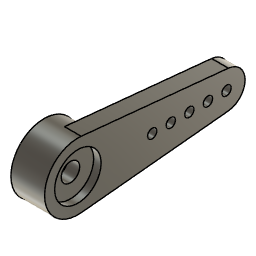
Servo half arm v1 (Autodesk Fusion 360 design; units mm, degrees)
Autodesk Fusion 360 part; units mm, degrees
note: some values were not read from the file. Set by a fixed rule: which sketch regions a step uses.
sketch "Sketch1" plane through (0, 0, 0) normal (1, 0, 0) x (0, 1, 0)
  circle A0 centre (0, 0) radius 3.58
  circle A1 centre (16, 0) radius 2
  line L0 (0.3535, 3.5625) -> (16.1975, 1.9902)
  line L1 (0.3535, -3.5625) -> (16.1975, -1.9902)
  circle A2 centre (16, 0) radius 0.5
  circle A3 centre (14, 0) radius 0.5
  circle A4 centre (12, 0) radius 0.5
  circle A5 centre (10, 0) radius 0.5
  circle A6 centre (8, 0) radius 0.5
  line L2 (0, 7) -> (0, -7.5)
  circle A7 centre (-8, 0) radius 0.5
  circle A8 centre (-10, 0) radius 0.5
  line L3 (-0.3535, 3.5625) -> (-16.1975, 1.9902)
  circle A9 centre (-12, 0) radius 0.5
  circle A10 centre (-14, 0) radius 0.5
  circle A11 centre (-16, 0) radius 2
  circle A12 centre (-16, 0) radius 0.5
  line L4 (-0.3535, -3.5625) -> (-16.1975, -1.9902)
  dimension "d4" = 7.16
  dimension "d5" = 4
  dimension "d6" = 16
  dimension "d7" = 1
  dimension "d10" = -8
  dimension "d11" = 0
  constraint coincident A0.centre origin
  constraint coincident A0 L0.start
  constraint coincident A1 L0.end
  constraint coincident A0 L1.start
  constraint coincident A1 L1.end
  constraint tangent A0 L0
  constraint tangent A1 L0
  constraint tangent A1 L1
  constraint tangent A0 L1
  constraint concentric A1 A2
  constraint vertical L2
  constraint coincident A0.centre L2
  constraint symmetric A1 L2 A11
  constraint symmetric L0.start L2 L3.start
  constraint symmetric L0.end L2 L3.end
  constraint symmetric L1.start L2 L4.start
  constraint symmetric L1.end L2 L4.end
  constraint symmetric A2 L2 A12
  constraint symmetric A3 L2 A10
  constraint symmetric A4 L2 A9
  constraint symmetric A5 L2 A8
  constraint symmetric A6 L2 A7
  measures "d4" diameter of A0
  measures "d5" diameter of A1
  measures "d6" distance of A0.centre A1.centre
  measures "d7" diameter of A2
extrude "Extrude1" add sketch "Sketch1" along normal blind 1.8 contours A0 L2 | A0 A1 L0 L1 A3 | A0 L2 | A1 A3 | A0 L3 A10 A11 L4 | A10 A11 picked at (14.8153, -0.6023) picked at (-14.8153, -0.6023) makes body 1
extrude "Extrude2" add sketch "Sketch1" along normal blind 1.8 separate body contours A0 L2 | A0 A1 L0 L1 A3 | A0 L2 | A1 A3 picked at (14.8153, -0.6023) makes body 2
sketch "Sketch2" plane through (0, 0, 0) normal (1, 0, 0) x (0, 1, 0)
extrude "Extrude3" add sketch "Sketch1" against normal blind 1.83 contours A0 L2 | A0 L2 bodies 1
sketch "Sketch3" plane through (1.8, 0, 0) normal (1, 0, 0) x (0, 1, 0)
  circle A0 centre (-10, 0) radius 0.5
  circle A1 centre (10, 0) radius 0.5
  circle A2 centre (-12, 0) radius 0.5
  circle A3 centre (12, 0) radius 0.5
  circle A4 centre (-8, 0) radius 0.5
  circle A5 centre (16, 0) radius 0.5
  circle A6 centre (-16, 0) radius 0.5
  circle A7 centre (14, 0) radius 0.5
  circle A8 centre (8, 0) radius 0.5
  circle A9 centre (-14, 0) radius 0.5
  line L0 (0.3535, -3.5625) -> (16.1975, -1.9902)
  arc A10 (16.1975, -1.9902) -> (16.1975, 1.9902) centre (16, 0) ccw
  line L1 (16.1975, 1.9902) -> (0.3535, 3.5625)
  arc A11 (0.3535, 3.5625) -> (-0.3535, 3.5625) centre (0, 0) ccw
  line L2 (-0.3535, 3.5625) -> (-16.1975, 1.9902)
  arc A12 (-16.1975, 1.9902) -> (-16.1975, -1.9902) centre (-16, 0) ccw
  line L3 (-16.1975, -1.9902) -> (-0.3535, -3.5625)
  arc A13 (-0.3535, -3.5625) -> (0.3535, -3.5625) centre (0, 0) ccw
  circle A14 centre (0, 0) radius 2.5
  circle A15 centre (0, 0) radius 3.58
  dimension "d18" = 5
  constraint concentric A14 A15
  measures "d18" diameter of A14
extrude "Extrude4" cut sketch "Sketch3" against normal blind 0.8 contours A14 bodies 1
sketch "Sketch4" plane through (1, 0, 0) normal (1, 0, 0) x (0, 1, 0)
  circle A0 centre (0, 0) radius 2.5
  circle A1 centre (0, 0) radius 2.5
  circle A2 centre (0, 0) radius 1
  dimension "d21" = 2
  constraint concentric A0 A1
  constraint concentric A1 A2
  measures "d21" diameter of A2
extrude "Extrude5" cut sketch "Sketch4" against normal blind 13.5 contours A2 bodies 1
sketch "Sketch5" plane through (-1.83, 0, 0) normal (-1, 0, 0) x (0, -1, 0)
  circle A0 centre (0, 0) radius 1
  circle A1 centre (0, 0) radius 3.58
  circle A2 centre (0, 0) radius 2.3
  dimension "d24" = 4.6
  constraint concentric A0 A2
  measures "d24" diameter of A2
extrude "Extrude6" cut sketch "Sketch5" against normal blind 1.5 contours A2 bodies 1
extrude "Extrude7" add sketch "Sketch1" against normal blind 1.83 contours A0 L2 | A0 L2 bodies 2
extrude "Extrude8" cut sketch "Sketch3" against normal blind 0.8 contours A14 bodies 2
extrude "Extrude9" cut sketch "Sketch5" against normal blind 1.5 contours A2 bodies 2
extrude "Extrude10" cut 1 faces at (-1.83, 0.6188, -0.2429) along direction (1, 0, 0) blind 27.5 on bodies 2 bodies 2
hidden bodies 1
equation "d4 = 3.58 * 2 mm"
equation "d16 = -3.43 mm + 1.6 mm"
equation "d27 = -3.43 mm + 1.6 mm"
named bodies: "2Horn", "1Horn"
